Autodesk Fusion 360 part; units mm, degrees
note: some values were not read from the file. Set by a fixed rule: which sketch regions a step uses.
(part 3 of 4)
extrude "Extrude2" add sketch "Sketch2" along normal blind 1.6 contours L4 L5 L6 L7 | L8 L9 L10 L11 | L12 L13 L14 L15 | L16 L17 L18 L19 | L20 L21 L22 L23 | L24 L25 L26 L27 | L28 L29 L30 L31 | L32 L33 L34 L35 | L36 L37 L38 L39 | L40 L41 L42 L43 | L44 L45 L46 L47 | L48 L49 L50 L51 | L52 L53 L54 L55 | L56 L57 L58 L59 | L60 L61 L62 L63 | L64 L65 L66 L67 | L68 L69 L70 L71 | L72 L73 L74 L75 | L76 L77 L78 L79 | L80 L81 L82 L83 | L84 L85 L86 L87 | L88 L89 L90 L91 | L92 L93 L94 L95 | L96 L97 L98 L99 | L100 L101 L102 L103 | L104 L105 L106 L107 | L108 L109 L110 L111 | L112 L113 L114 L115 | L116 L117 L118 L119 | L120 L121 L122 L123 | L124 L125 L126 L127 | L128 L129 L130 L131 | L132 L133 L134 L135 | L136 L137 L138 L139 | L140 L141 L142 L143 | L144 L145 L146 L147 | L148 L149 L150 L151 | L152 L153 L154 L155 | L156 L157 L158 L159 | L160 L161 L162 L163 | L164 L165 L166 L167 | L168 L169 L170 L171 | L172 L173 L174 L175 | L176 L177 L178 L179 | L180 L181 L182 L183 | L184 L185 L186 L187 | L188 L189 L190 L191 | L192 L193 L194 L195 | L196 L197 L198 L199 | L200 L201 L202 L203 | L204 L205 L206 L207 | L208 L209 L210 L211 | L212 L213 L214 L215 | L216 L217 L218 L219 | L220 L221 L222 L223 | L224 L225 L226 L227 | L228 L229 L230 L231 | L232 L233 L234 L235 | L236 L237 L238 L239 | L240 L241 L242 L243 | L244 L245 L246 L247 | L248 L249 L250 L251 | L252 L253 L254 L255 | L256 L257 L258 L259 | L260 L261 L262 L263 | L264 L265 L266 L267 | L268 L269 L270 L271 | L272 L273 L274 L275 | L276 L277 L278 L279 | L280 L281 L282 L283 | L284 L285 L286 L287 | L288 L289 L290 L291 | L292 L293 L294 L295 | L296 L297 L298 L299 | L300 L301 L302 L303 | L304 L305 L306 L307 | L308 L309 L310 L311 | L312 L313 L314 L315 | L316 L317 L318 L319 | L320 L321 L322 L323 | L324 L325 L326 L327 | L328 L329 L330 L331 | L332 L333 L334 L335 | L336 L337 L338 L339 | L340 L341 L342 L343 | L344 L345 L346 L347 | L348 L349 L350 L351 | L352 L353 L354 L355 | L356 L357 L358 L359 | L360 L361 L362 L363 | L364 L365 L366 L367 | L368 L369 L370 L371 | L372 L373 L374 L375 | L376 L377 L378 L379 | L380 L381 L382 L383 | L384 L385 L386 L387 | L388 L389 L390 L391 | L392 L393 L394 L395 | L396 L397 L398 L399 | L400 L401 L402 L403 | L404 L405 L406 L407 | L408 L409 L410 L411 | L412 L413 L414 L415 | L416 L417 L418 L419 | L420 L421 L422 L423 | L424 L425 L426 L427 | L428 L429 L430 L431 | L432 L433 L434 L435 | L436 L437 L438 L439 | L440 L441 L442 L443 | L444 L445 L446 L447 | L448 L449 L450 L451 | L452 L453 L454 L455 | L456 L457 L458 L459 | L460 L461 L462 L463 | L464 L465 L466 L467 | L468 L469 L470 L471 | L472 L473 L474 L475 | L476 L477 L478 L479 | L480 L481 L482 L483 | L484 L485 L486 L487 | L488 L489 L490 L491 | L492 L493 L494 L495 | L496 L497 L498 L499 | L500 L501 L502 L503 | L504 L505 L506 L507 | L508 L509 L510 L511 | L512 L513 L514 L515 | L516 L517 L518 L519 | L520 L521 L522 L523 | L524 L525 L526 L527 | L528 L529 L530 L531 | L532 L533 L534 L535 | L536 L537 L538 L539 | L540 L541 L542 L543 | L544 L545 L546 L547 | L548 L549 L550 L551 | L552 L553 L554 L555 | L556 L557 L558 L559 | L560 L561 L562 L563 | L564 L565 L566 L567 | L568 L569 L570 L571 | L572 L573 L574 L575 | L576 L577 L578 L579 | L580 L581 L582 L583 | L584 L585 L586 L587 | L588 L589 L590 L591 | L592 L593 L594 L595 | L596 L597 L598 L599 | L600 L601 L602 L603 | L604 L605 L606 L607 | L608 L609 L610 L611 | L612 L613 L614 L615 | L616 L617 L618 L619 | L620 L621 L622 L623 | L624 L625 L626 L627 | L628 L629 L630 L631 | L632 L633 L634 L635 | L636 L637 L638 L639 | L640 L641 L642 L643 | L644 L645 L646 L647 | L648 L649 L650 L651 | L652 L653 L654 L655 | L656 L657 L658 L659 | L660 L661 L662 L663 | L664 L665 L666 L667 | L668 L669 L670 L671 | L672 L673 L674 L675 | L676 L677 L678 L679 | L680 L681 L682 L683 | L684 L685 L686 L687 | L688 L689 L690 L691 | L692 L693 L694 L695 | L696 L697 L698 L699 | L700 L701 L702 L703 | L704 L705 L706 L707 | L708 L709 L710 L711 | L712 L713 L714 L715 | L716 L717 L718 L719 | L720 L721 L722 L723 | L724 L725 L726 L727 | L728 L729 L730 L731 | L732 L733 L734 L735 | L736 L737 L738 L739 | L740 L741 L742 L743 | L744 L745 L746 L747 | L748 L749 L750 L751 | L752 L753 L754 L755 | L756 L757 L758 L759 | L760 L761 L762 L763 | L764 L765 L766 L767 | L768 L769 L770 L771 | L772 L773 L774 L775 | L776 L777 L778 L779 | L780 L781 L782 L783 | L784 L785 L786 L787 | L788 L789 L790 L791 | L792 L793 L794 L795 | L796 L797 L798 L799 | L800 L801 L802 L803 | L804 L805 L806 L807 | L808 L809 L810 L811 | L812 L813 L814 L815 | L816 L817 L818 L819 | L820 L821 L822 L823 | L824 L825 L826 L827 | L828 L829 L830 L831 | L832 L833 L834 L835 | L836 L837 L838 L839 | L840 L841 L842 L843 | L844 L845 L846 L847 | L848 L849 L850 L851 | L852 L853 L854 L855 | L856 L857 L858 L859 | L860 L861 L862 L863 | L864 L865 L866 L867 | L868 L869 L870 L871 | L872 L873 L874 L875 | L876 L877 L878 L879 | L880 L881 L882 L883 | L884 L885 L886 L887 | L888 L889 L890 L891 | L892 L893 L894 L895 | L896 L897 L898 L899 | L900 L901 L902 L903 | L904 L905 L906 L907 | L908 L909 L910 L911 | L912 L913 L914 L915 | L916 L917 L918 L919 | L920 L921 L922 L923 | L924 L925 L926 L927 | L928 L929 L930 L931 | L932 L933 L934 L935 | L936 L937 L938 L939 | L940 L941 L942 L943 | L944 L945 L946 L947 | L948 L949 L950 L951 | L952 L953 L954 L955 | L956 L957 L958 L959 | L960 L961 L962 L963 | L964 L965 L966 L967 | L968 L969 L970 L971 | L972 L973 L974 L975 | L976 L977 L978 L979 | L980 L981 L982 L983 | L984 L985 L986 L987 | L988 L989 L990 L991 | L992 L993 L994 L995 | L996 L997 L998 L999 | L1000 L1001 L1002 L1003 | L1004 L1005 L1006 L1007 | L1008 L1009 L1010 L1011 | L1012 L1013 L1014 L1015 | L1016 L1017 L1018 L1019 | L1020 L1021 L1022 L1023 | L1024 L1025 L1026 L1027 bodies 1 in component "LED_Pannel"
extrude "Extrude3" add sketch "Sketch2" along normal blind 1 contours L1028 L1029 L1030 L1031 | L1032 L1033 L1034 L1035 | L1036 L1037 L1038 L1039 | L1040 L1041 L1042 L1043 | L1044 L1045 L1046 L1047 | L1048 L1049 L1050 L1051 | L1052 L1053 L1054 L1055 | L1056 L1057 L1058 L1059 | L1060 L1061 L1062 L1063 | L1064 L1065 L1066 L1067 | L1068 L1069 L1070 L1071 | L1072 L1073 L1074 L1075 | L1076 L1077 L1078 L1079 | L1080 L1081 L1082 L1083 | L1084 L1085 L1086 L1087 | L1088 L1089 L1090 L1091 | L1092 L1093 L1094 L1095 | L1096 L1097 L1098 L1099 | L1100 L1101 L1102 L1103 | L1104 L1105 L1106 L1107 | L1108 L1109 L1110 L1111 | L1112 L1113 L1114 L1115 | L1116 L1117 L1118 L1119 | L1120 L1121 L1122 L1123 | L1124 L1125 L1126 L1127 | L1128 L1129 L1130 L1131 | L1132 L1133 L1134 L1135 | L1136 L1137 L1138 L1139 | L1140 L1141 L1142 L1143 | L1144 L1145 L1146 L1147 | L1148 L1149 L1150 L1151 | L1152 L1153 L1154 L1155 | L1156 L1157 L1158 L1159 | L1160 L1161 L1162 L1163 | L1164 L1165 L1166 L1167 | L1168 L1169 L1170 L1171 | L1172 L1173 L1174 L1175 | L1176 L1177 L1178 L1179 | L1180 L1181 L1182 L1183 | L1184 L1185 L1186 L1187 | L1188 L1189 L1190 L1191 | L1192 L1193 L1194 L1195 | L1196 L1197 L1198 L1199 | L1200 L1201 L1202 L1203 | L1204 L1205 L1206 L1207 | L1208 L1209 L1210 L1211 | L1212 L1213 L1214 L1215 | L1216 L1217 L1218 L1219 | L1220 L1221 L1222 L1223 | L1224 L1225 L1226 L1227 | L1228 L1229 L1230 L1231 | L1232 L1233 L1234 L1235 | L1236 L1237 L1238 L1239 | L1240 L1241 L1242 L1243 | L1244 L1245 L1246 L1247 | L1248 L1249 L1250 L1251 | L1252 L1253 L1254 L1255 | L1256 L1257 L1258 L1259 | L1260 L1261 L1262 L1263 | L1264 L1265 L1266 L1267 | L1268 L1269 L1270 L1271 | L1272 L1273 L1274 L1275 | L1276 L1277 L1278 L1279 | L1280 L1281 L1282 L1283 | L1284 L1285 L1286 L1287 | L1288 L1289 L1290 L1291 | L1292 L1293 L1294 L1295 | L1296 L1297 L1298 L1299 | L1300 L1301 L1302 L1303 | L1304 L1305 L1306 L1307 | L1308 L1309 L1310 L1311 | L1312 L1313 L1314 L1315 | L1316 L1317 L1318 L1319 | L1320 L1321 L1322 L1323 | L1324 L1325 L1326 L1327 | L1328 L1329 L1330 L1331 | L1332 L1333 L1334 L1335 | L1336 L1337 L1338 L1339 | L1340 L1341 L1342 L1343 | L1344 L1345 L1346 L1347 | L1348 L1349 L1350 L1351 | L1352 L1353 L1354 L1355 | L1356 L1357 L1358 L1359 | L1360 L1361 L1362 L1363 | L1364 L1365 L1366 L1367 | L1368 L1369 L1370 L1371 | L1372 L1373 L1374 L1375 | L1376 L1377 L1378 L1379 | L1380 L1381 L1382 L1383 | L1384 L1385 L1386 L1387 | L1388 L1389 L1390 L1391 | L1392 L1393 L1394 L1395 | L1396 L1397 L1398 L1399 | L1400 L1401 L1402 L1403 | L1404 L1405 L1406 L1407 | L1408 L1409 L1410 L1411 | L1412 L1413 L1414 L1415 | L1416 L1417 L1418 L1419 | L1420 L1421 L1422 L1423 | L1424 L1425 L1426 L1427 | L1428 L1429 L1430 L1431 | L1432 L1433 L1434 L1435 | L1436 L1437 L1438 L1439 | L1440 L1441 L1442 L1443 | L1444 L1445 L1446 L1447 | L1448 L1449 L1450 L1451 | L1452 L1453 L1454 L1455 | L1456 L1457 L1458 L1459 | L1460 L1461 L1462 L1463 | L1464 L1465 L1466 L1467 | L1468 L1469 L1470 L1471 | L1472 L1473 L1474 L1475 | L1476 L1477 L1478 L1479 | L1480 L1481 L1482 L1483 | L1484 L1485 L1486 L1487 | L1488 L1489 L1490 L1491 | L1492 L1493 L1494 L1495 | L1496 L1497 L1498 L1499 | L1500 L1501 L1502 L1503 | L1504 L1505 L1506 L1507 | L1508 L1509 L1510 L1511 | L1512 L1513 L1514 L1515 | L1516 L1517 L1518 L1519 | L1520 L1521 L1522 L1523 | L1524 L1525 L1526 L1527 | L1528 L1529 L1530 L1531 | L1532 L1533 L1534 L1535 | L1536 L1537 L1538 L1539 | L1540 L1541 L1542 L1543 | L1544 L1545 L1546 L1547 | L1548 L1549 L1550 L1551 | L1552 L1553 L1554 L1555 | L1556 L1557 L1558 L1559 | L1560 L1561 L1562 L1563 | L1564 L1565 L1566 L1567 | L1568 L1569 L1570 L1571 | L1572 L1573 L1574 L1575 | L1576 L1577 L1578 L1579 | L1580 L1581 L1582 L1583 | L1584 L1585 L1586 L1587 | L1588 L1589 L1590 L1591 | L1592 L1593 L1594 L1595 | L1596 L1597 L1598 L1599 | L1600 L1601 L1602 L1603 | L1604 L1605 L1606 L1607 | L1608 L1609 L1610 L1611 | L1612 L1613 L1614 L1615 | L1616 L1617 L1618 L1619 | L1620 L1621 L1622 L1623 | L1624 L1625 L1626 L1627 | L1628 L1629 L1630 L1631 | L1632 L1633 L1634 L1635 | L1636 L1637 L1638 L1639 | L1640 L1641 L1642 L1643 | L1644 L1645 L1646 L1647 | L1648 L1649 L1650 L1651 | L1652 L1653 L1654 L1655 | L1656 L1657 L1658 L1659 | L1660 L1661 L1662 L1663 | L1664 L1665 L1666 L1667 | L1668 L1669 L1670 L1671 | L1672 L1673 L1674 L1675 | L1676 L1677 L1678 L1679 | L1680 L1681 L1682 L1683 | L1684 L1685 L1686 L1687 | L1688 L1689 L1690 L1691 | L1692 L1693 L1694 L1695 | L1696 L1697 L1698 L1699 | L1700 L1701 L1702 L1703 | L1704 L1705 L1706 L1707 | L1708 L1709 L1710 L1711 | L1712 L1713 L1714 L1715 | L1716 L1717 L1718 L1719 | L1720 L1721 L1722 L1723 | L1724 L1725 L1726 L1727 | L1728 L1729 L1730 L1731 | L1732 L1733 L1734 L1735 | L1736 L1737 L1738 L1739 | L1740 L1741 L1742 L1743 | L1744 L1745 L1746 L1747 | L1748 L1749 L1750 L1751 | L1752 L1753 L1754 L1755 | L1756 L1757 L1758 L1759 | L1760 L1761 L1762 L1763 | L1764 L1765 L1766 L1767 | L1768 L1769 L1770 L1771 | L1772 L1773 L1774 L1775 | L1776 L1777 L1778 L1779 | L1780 L1781 L1782 L1783 | L1784 L1785 L1786 L1787 | L1788 L1789 L1790 L1791 | L1792 L1793 L1794 L1795 | L1796 L1797 L1798 L1799 | L1800 L1801 L1802 L1803 | L1804 L1805 L1806 L1807 | L1808 L1809 L1810 L1811 | L1812 L1813 L1814 L1815 | L1816 L1817 L1818 L1819 | L1820 L1821 L1822 L1823 | L1824 L1825 L1826 L1827 | L1828 L1829 L1830 L1831 | L1832 L1833 L1834 L1835 | L1836 L1837 L1838 L1839 | L1840 L1841 L1842 L1843 | L1844 L1845 L1846 L1847 | L1848 L1849 L1850 L1851 | L1852 L1853 L1854 L1855 | L1856 L1857 L1858 L1859 | L1860 L1861 L1862 L1863 | L1864 L1865 L1866 L1867 | L1868 L1869 L1870 L1871 | L1872 L1873 L1874 L1875 | L1876 L1877 L1878 L1879 | L1880 L1881 L1882 L1883 | L1884 L1885 L1886 L1887 | L1888 L1889 L1890 L1891 | L1892 L1893 L1894 L1895 | L1896 L1897 L1898 L1899 | L1900 L1901 L1902 L1903 | L1904 L1905 L1906 L1907 | L1908 L1909 L1910 L1911 | L1912 L1913 L1914 L1915 | L1916 L1917 L1918 L1919 | L1920 L1921 L1922 L1923 | L1924 L1925 L1926 L1927 | L1928 L1929 L1930 L1931 | L1932 L1933 L1934 L1935 | L1936 L1937 L1938 L1939 | L1940 L1941 L1942 L1943 | L1944 L1945 L1946 L1947 | L1948 L1949 L1950 L1951 | L1952 L1953 L1954 L1955 | L1956 L1957 L1958 L1959 | L1960 L1961 L1962 L1963 | L1964 L1965 L1966 L1967 | L1968 L1969 L1970 L1971 | L1972 L1973 L1974 L1975 | L1976 L1977 L1978 L1979 | L1980 L1981 L1982 L1983 | L1984 L1985 L1986 L1987 bodies 1 in component "LED_Pannel"
sketch "Sketch1 (2)" plane through (0, 0, 0) normal (0, 0, 1) x (1, 0, 0) in component "Diffusion"
  line L0 (0, 0) -> (170, 0)
  line L1 (170, 0) -> (170, 170)
  line L2 (170, 170) -> (0, 170)
  line L3 (0, 170) -> (0, 0)
  dimension "d26" = 170
  constraint horizontal L0
  constraint vertical L1
  constraint horizontal L2
  constraint vertical L3
  constraint coincident L0.start L3.end
  constraint equal L2 L3
  measures "d26" distance of L0.start L2.end
extrude "Extrude1'" add sketch "Sketch1 (2)" along normal blind 3 separate body makes body 2 in component "Diffusion"
sketch "Sketch1 (3)" plane through (0, 0, 0) normal (0, 0, 1) x (1, 0, 0) in component "Backing"
  line L0 (0, 0) -> (170, 0)
  line L1 (170, 0) -> (170, 170)
  line L2 (170, 170) -> (0, 170)
  line L3 (0, 170) -> (0, 0)
  dimension "d26_1" = 170
  constraint horizontal L0
  constraint vertical L1
  constraint horizontal L2
  constraint vertical L3
  constraint coincident L0.start L3.end
  constraint equal L2 L3
  measures "d26_1" distance of L0.start L2.end
extrude "Extrude1''" add sketch "Sketch1 (3)" along normal blind 3 separate body makes body 3 in component "Backing"
sketch "Sketch1 (4)" plane through (0, 0, 0) normal (0, 0, 1) x (1, 0, 0) in component "Side(holes)"
  line L0 (0, 0) -> (180, 0)
  line L1 (180, 0) -> (180, 54)
  line L2 (180, 54) -> (0, 54)
  line L3 (0, 54) -> (0, 0)
  line L4 (175, 54) -> (175, 0) construction
  line L5 (5, 54) -> (5, 0) construction
  line L6 (0, 27) -> (180, 27) construction
  circle A0 centre (5, 43) radius 1.6
  circle A1 centre (5, 11) radius 1.6
  circle A2 centre (175, 43) radius 1.6
  circle A3 centre (175, 11) radius 1.6
  line L7 (5, 48) -> (175, 48) construction
  line L8 (175, 48) -> (175, 51) construction
  line L9 (175, 51) -> (5, 51) construction
  line L10 (5, 51) -> (5, 48) construction
  line L11 (5, 3) -> (175, 3) construction
  line L12 (175, 3) -> (175, 6) construction
  line L13 (175, 6) -> (5, 6) construction
  line L14 (5, 6) -> (5, 3) construction
  line L15 (90, 54) -> (90, 0) construction
  line L16 (10, 36) -> (170, 36) construction
  line L17 (170, 36) -> (170, 48) construction
  line L18 (170, 48) -> (10, 48) construction
  line L19 (10, 48) -> (10, 36) construction
  point P0 (90, 48)
  point P1 (90, 6)
  point P2 (90, 48)
  dimension "d31" = 5
  dimension "d32" = 5
  dimension "d34" = 3.2
  dimension "d36" = 3.2
  dimension "d37" = 3.2
  dimension "d38" = 3.2
  dimension "d68" = 170
  dimension "d69" = 3
  dimension "d70" = 3
  dimension "d71" = 170
  dimension "d72" = 3
  dimension "d73" = 3
  dimension "d74" = 12
  dimension "d75" = 160
  dimension "d76" = 30
  dimension "d77" = 10
  dimension "d78" = 5
  dimension "d79" = 5
  dimension "d80" = 5
  dimension "d81" = 5
  constraint horizontal L0
  constraint vertical L1
  constraint horizontal L2
  constraint vertical L3
  constraint coincident L0.start L3.end
  constraint coincident L2 L4.start
  constraint coincident L0 L4.end
  constraint perpendicular L0 L4
  constraint coincident L2 L5.start
  constraint coincident L0 L5.end
  constraint perpendicular L0 L5
  constraint midpoint L3 L6.start
  constraint midpoint L1 L6.end
  constraint coincident L5 A0.centre
  constraint coincident L5 A1.centre
  constraint coincident L4 A2.centre
  constraint coincident L4 A3.centre
  constraint horizontal L7
  constraint vertical L8
  constraint horizontal L9
  constraint vertical L10
  constraint horizontal L11
  constraint vertical L12
  constraint horizontal L13
  constraint vertical L14
  constraint midpoint L2 L15.start
  constraint midpoint L0 L15.end
  constraint midpoint L7 P2
  constraint midpoint L13 P1
  constraint coincident L15 P1
  constraint coincident L15 P2
  constraint horizontal L16
  constraint vertical L17
  constraint horizontal L18
  constraint vertical L19
  constraint midpoint L18 P2
  constraint coincident P2 P0
  measures "d31" distance of L3 L5
  measures "d32" distance of L1 L4
  measures "d34" diameter of A0
  measures "d36" diameter of A1
  measures "d37" diameter of A2
  measures "d38" diameter of A3
  measures "d68" distance of L7.start L7.end
  measures "d69" distance of L7.start L9.end
  measures "d70" distance of L11.start L13.end
  measures "d71" distance of L12.end L13.end
  measures "d72" distance of L2 L9
  measures "d73" distance of L0 L11
  measures "d74" distance of L16.start L18.end
  measures "d75" distance of L17.end L18.end
  measures "d76" distance of L13 L16
  measures "d77" distance of L3 L19
  measures "d78" distance of A0.centre L7
  measures "d79" distance of A1.centre L13
  measures "d80" distance of A2.centre L7.end
  measures "d81" distance of A3.centre L12.end
extrude "Extrude1'''" add sketch "Sketch1 (4)" along normal blind 10 separate body makes body 4 in component "Side(holes)"
sketch "Sketch2 (2)" plane through (0, 0, 10) normal (0, 0, 1) x (-1, 0, 0) in component "Side(holes)"
  circle A0 centre (-5, -43) radius 1.6 construction
  circle A1 centre (-175, -43) radius 1.6 construction
  circle A2 centre (-5, -11) radius 1.6 construction
  circle A3 centre (-175, -11) radius 1.6 construction
  line L0 (0, -54) -> (0, 0) construction
  line L1 (0, 0) -> (-180, 0) construction
  line L2 (-180, 0) -> (-180, -54) construction
  line L3 (-180, -54) -> (0, -54) construction
  line L4 (-5, -48) -> (-175, -48)
  line L5 (-175, -48) -> (-175, -51)
  line L6 (-175, -51) -> (-5, -51)
  line L7 (-5, -51) -> (-5, -48)
  line L8 (-90, -54) -> (-90, 0) construction
  line L9 (-5, -6) -> (-175, -6)
  line L10 (-175, -6) -> (-175, -3)
  line L11 (-175, -3) -> (-5, -3)
  line L12 (-5, -3) -> (-5, -6)
  line L13 (-89, -48) -> (-91, -48)
  line L14 (-91, -48) -> (-91, -38)
  line L15 (-91, -38) -> (-89, -38)
  line L16 (-89, -38) -> (-89, -48)
  line L17 (-159, -38) -> (-159, -48)
  line L18 (-161, -48) -> (-161, -38)
  line L19 (-161, -38) -> (-159, -38)
  line L20 (-149, -38) -> (-149, -48)
  line L21 (-151, -48) -> (-151, -38)
  line L22 (-151, -38) -> (-149, -38)
  line L23 (-139, -38) -> (-139, -48)
  line L24 (-141, -48) -> (-141, -38)
  line L25 (-141, -38) -> (-139, -38)
  line L26 (-129, -38) -> (-129, -48)
  line L27 (-131, -48) -> (-131, -38)
  line L28 (-131, -38) -> (-129, -38)
  line L29 (-119, -38) -> (-119, -48)
  line L30 (-121, -48) -> (-121, -38)
  line L31 (-121, -38) -> (-119, -38)
  line L32 (-109, -38) -> (-109, -48)
  line L33 (-111, -48) -> (-111, -38)
  line L34 (-111, -38) -> (-109, -38)
  line L35 (-99, -38) -> (-99, -48)
  line L36 (-101, -48) -> (-101, -38)
  line L37 (-101, -38) -> (-99, -38)
  line L38 (-79, -38) -> (-79, -48)
  line L39 (-81, -48) -> (-81, -38)
  line L40 (-81, -38) -> (-79, -38)
  line L41 (-69, -38) -> (-69, -48)
  line L42 (-71, -48) -> (-71, -38)
  line L43 (-71, -38) -> (-69, -38)
  line L44 (-59, -38) -> (-59, -48)
  line L45 (-61, -48) -> (-61, -38)
  line L46 (-61, -38) -> (-59, -38)
  line L47 (-49, -38) -> (-49, -48)
  line L48 (-51, -48) -> (-51, -38)
  line L49 (-51, -38) -> (-49, -38)
  line L50 (-39, -38) -> (-39, -48)
  line L51 (-41, -48) -> (-41, -38)
  line L52 (-41, -38) -> (-39, -38)
  line L53 (-29, -38) -> (-29, -48)
  line L54 (-31, -48) -> (-31, -38)
  line L55 (-31, -38) -> (-29, -38)
  line L56 (-19, -38) -> (-19, -48)
  line L57 (-21, -48) -> (-21, -38)
  line L58 (-21, -38) -> (-19, -38)
  line L59 (-10, -48) -> (-10, -36)
  line L60 (-10, -36) -> (-170, -36)
  line L61 (-170, -36) -> (-170, -48)
  line L62 (-180, -21) -> (0, -21) construction
  line L63 (-10, -36) -> (-10, -6) construction
  line L64 (-170, -36) -> (-170, -6) construction
  circle A4 centre (-25.85, -21) radius 3.85
  circle A5 centre (-44.55, -21) radius 2.85
  circle A6 centre (-65.4, -21) radius 6
  line L65 (-18.35, -28.5) -> (-33.35, -28.5)
  line L66 (-33.35, -28.5) -> (-33.35, -13.5)
  line L67 (-33.35, -13.5) -> (-18.35, -13.5)
  line L68 (-18.35, -13.5) -> (-18.35, -28.5)
  line L69 (-34.55, -31) -> (-54.55, -31)
  line L70 (-54.55, -31) -> (-54.55, -11)
  line L71 (-54.55, -11) -> (-34.55, -11)
  line L72 (-34.55, -11) -> (-34.55, -31)
  line L73 (-57.4, -29) -> (-73.4, -29)
  line L74 (-73.4, -29) -> (-73.4, -13)
  line L75 (-73.4, -13) -> (-57.4, -13)
  line L76 (-57.4, -13) -> (-57.4, -29)
  line L77 (-73.4, -29) -> (-57.4, -13) construction
  line L78 (-54.55, -31) -> (-34.55, -11) construction
  line L79 (-33.35, -28.5) -> (-18.35, -13.5) construction
  point P0 (-90, -51)
  point P1 (-90, -6)
  point P2 (-90, -38)
  point P3 (-90, -48)
  point P4 (-90, -38)
  point P5 (-10, -21)
  point P6 (-10, -21)
  point P7 (-170, -21)
  point P8 (-29.7, -21)
  point P9 (-41.7, -21)
  point P10 (-47.4, -21)
  point P11 (-59.4, -21)
  point P12 (-71.4, -21)
  point P13 (-22, -21)
  point P14 (-25.85, -21)
  point P15 (-44.55, -21)
  point P16 (-65.4, -21)
  dimension "d44" = 170
  dimension "d45" = 3
  dimension "d46" = 3
  dimension "d47" = 170
  dimension "d48" = 3
  dimension "d49" = 3
  dimension "d50" = 2
  dimension "d51" = 10
  dimension "d54" = 10
  dimension "d55" = 0
  dimension "d83" = 7.7
  dimension "d84" = 5.7
  dimension "d85" = 12
  dimension "d87" = 12
  dimension "d88" = 12
  dimension "d89" = 12
  dimension "d93" = 16
  dimension "d94" = 20
  dimension "d95" = 15
  constraint horizontal L4
  constraint vertical L5
  constraint horizontal L6
  constraint vertical L7
  constraint midpoint L3 L8.start
  constraint midpoint L1 L8.end
  constraint midpoint L6 P0
  constraint coincident L8 P0
  constraint horizontal L9
  constraint vertical L10
  constraint horizontal L11
  constraint vertical L12
  constraint midpoint L9 P1
  constraint coincident L8 P1
  constraint horizontal L13
  constraint vertical L14
  constraint horizontal L15
  constraint vertical L16
  constraint midpoint L15 P4
  constraint coincident L8 P4
  constraint midpoint L13 P3
  constraint coincident L4 P3
  constraint coincident P4 P2
  constraint coincident L2 L62.start
  constraint coincident L0 L62.end
  constraint perpendicular L0 L62
  constraint coincident L59.end L60.start
  constraint coincident L9 L63.end
  constraint perpendicular L9 L63
  constraint midpoint L63 P6
  constraint coincident L62 P6
  constraint coincident P6 P5
  constraint coincident L60.end L61.start
  constraint coincident L9 L64.end
  constraint perpendicular L9 L64
  constraint midpoint L64 P7
  constraint coincident L62 P14
  constraint coincident L62 P15
  constraint coincident L62 P16
  constraint coincident A4 P8
  constraint coincident L62 P8
  constraint coincident A5 P9
  constraint coincident L62 P9
  constraint coincident A5 P10
  constraint coincident L62 P10
  constraint coincident A6 P11
  constraint coincident L62 P11
  constraint coincident A6 P12
  constraint coincident L62 P12
  constraint coincident A4 P13
  constraint coincident L62 P13
  constraint horizontal L65
  constraint vertical L66
  constraint horizontal L67
  constraint vertical L68
  constraint horizontal L69
  constraint vertical L70
  constraint horizontal L71
  constraint vertical L72
  constraint horizontal L73
  constraint vertical L74
  constraint horizontal L75
  constraint vertical L76
  constraint midpoint L79 P14
  constraint midpoint L78 P15
  constraint midpoint L77 P16
  constraint coincident P14 A4.centre
  constraint coincident P15 A5.centre
  constraint coincident P16 A6.centre
  constraint equal L65 L68
  constraint equal L69 L72
  constraint equal L73 L76
  measures "d44" distance of L4.start L4.end
  measures "d45" distance of L4.start L6.end
  measures "d46" distance of L3 L6
  measures "d47" distance of L9.start L9.end
  measures "d48" distance of L9.start L11.end
  measures "d49" distance of L1 L11
  measures "d50" distance of L13.start L13.end
  measures "d51" distance of L13.start L15.end
  measures "d83" diameter of A4
  measures "d84" diameter of A5
  measures "d85" diameter of A6
  measures "d87" distance of P6 P13
  measures "d88" distance of P8 P9
  measures "d89" distance of P10 P11
  measures "d93" distance of L74.end L75.end
  measures "d94" distance of L70.end L71.end
  measures "d95" distance of L66.end L67.end
extrude "Extrude2'" cut sketch "Sketch2 (2)" against normal blind 5 contours L4 L5 L6 L7 L13 | L4 L56 L57 L58 | L4 L53 L54 L55 | L4 L17 L18 L19 | L4 L50 L51 L52 | L4 L20 L21 L22 | L4 L47 L48 L49 | L4 L23 L24 L25 | L4 L44 L45 L46 | L4 L26 L27 L28 | L4 L41 L42 L43 | L4 L29 L30 L31 | L4 L38 L39 L40 | L4 L32 L33 L34 | L4 L13 L14 L15 L16 | L4 L35 L36 L37 | L9 L10 L11 L12 bodies 4 in component "Side(holes)"
chamfer "Chamfer2" distance 1 angle 45 66 edges at (5, 49.5, 10) (12, 48, 10) (19, 43, 10) (21, 43, 10) (20, 38, 10) (25, 48, 10) (29, 43, 10) (31, 43, 10) (30, 38, 10) (35, 48, 10) (41, 43, 10) (39, 43, 10) (40, 38, 10) (51, 43, 10) (49, 43, 10) (45, 48, 10) (50, 38, 10) (61, 43, 10) (59, 43, 10) (55, 48, 10) (60, 38, 10) (65, 48, 10) (69, 43, 10) (71, 43, 10) (70, 38, 10) (79, 43, 10) (81, 43, 10) (75, 48, 10) (80, 38, 10) (85, 48, 10) (89, 43, 10) (91, 43, 10) (90, 38, 10) (95, 48, 10) (99, 43, 10) (101, 43, 10) (100, 38, 10) (105, 48, 10) (109, 43, 10) (111, 43, 10) (110, 38, 10) (115, 48, 10) (119, 43, 10) (121, 43, 10) (120, 38, 10) (125, 48, 10) (129, 43, 10) (131, 43, 10) (130, 38, 10) (135, 48, 10) (139, 43, 10) (141, 43, 10) (140, 38, 10) (145, 48, 10) (149, 43, 10) (150, 38, 10) (151, 43, 10) (155, 48, 10) (159, 43, 10) (161, 43, 10) (160, 38, 10) (168, 48, 10) (175, 49.5, 10) (5, 4.5, 10) (90, 6, 10) (175, 4.5, 10) on bodies 4 in component "Side(holes)"
extrude "Extrude3'" cut sketch "Sketch2 (2)" against normal blind 10 contours A4 | A5 | A6 bodies 4 in component "Side(holes)"
extrude "Extrude4" cut sketch "Sketch2 (2)" against normal blind 8 contours L65 L66 L67 L68 | L69 L70 L71 L72 | L73 L74 L75 L76 bodies 4 in component "Side(holes)"
sketch "Sketch1 (5)" plane through (0, 0, 0) normal (0, 0, 1) x (1, 0, 0) in component "Side(no holes)"
  line L0 (0, 0) -> (180, 0)
  line L1 (180, 0) -> (180, 54)
  line L2 (180, 54) -> (0, 54)
  line L3 (0, 54) -> (0, 0)
  line L4 (175, 54) -> (175, 0) construction
  line L5 (5, 54) -> (5, 0) construction
  line L6 (0, 27) -> (180, 27) construction
  circle A0 centre (5, 43) radius 1.6
  circle A1 centre (5, 11) radius 1.6
  circle A2 centre (175, 43) radius 1.6
  circle A3 centre (175, 11) radius 1.6
  line L7 (5, 48) -> (175, 48) construction
  line L8 (175, 48) -> (175, 51) construction
  line L9 (175, 51) -> (5, 51) construction
  line L10 (5, 51) -> (5, 48) construction
  line L11 (5, 3) -> (175, 3) construction
  line L12 (175, 3) -> (175, 6) construction
  line L13 (175, 6) -> (5, 6) construction
  line L14 (5, 6) -> (5, 3) construction
  line L15 (90, 54) -> (90, 0) construction
  line L16 (10, 36) -> (170, 36) construction
  line L17 (170, 36) -> (170, 48) construction
  line L18 (170, 48) -> (10, 48) construction
  line L19 (10, 48) -> (10, 36) construction
  point P0 (90, 48)
  point P1 (90, 6)
  point P2 (90, 48)
  dimension "d31_1" = 5
  dimension "d32_1" = 5
  dimension "d34_1" = 3.2
  dimension "d36_1" = 3.2
  dimension "d37_1" = 3.2
  dimension "d38_1" = 3.2
  dimension "d68_1" = 170
  dimension "d69_1" = 3
  dimension "d70_1" = 3
  dimension "d71_1" = 170
  dimension "d72_1" = 3
  dimension "d73_1" = 3
  dimension "d74_1" = 12
  dimension "d75_1" = 160
  dimension "d76_1" = 30
  dimension "d77_1" = 10
  dimension "d78_1" = 5
  dimension "d79_1" = 5
  dimension "d80_1" = 5
  dimension "d81_1" = 5
  constraint horizontal L0
  constraint vertical L1
  constraint horizontal L2
  constraint vertical L3
  constraint coincident L0.start L3.end
  constraint coincident L2 L4.start
  constraint coincident L0 L4.end
  constraint perpendicular L0 L4
  constraint coincident L2 L5.start
  constraint coincident L0 L5.end
  constraint perpendicular L0 L5
  constraint midpoint L3 L6.start
  constraint midpoint L1 L6.end
  constraint coincident L5 A0.centre
  constraint coincident L5 A1.centre
  constraint coincident L4 A2.centre
  constraint coincident L4 A3.centre
  constraint horizontal L7
  constraint vertical L8
  constraint horizontal L9
  constraint vertical L10
  constraint horizontal L11
  constraint vertical L12
  constraint horizontal L13
  constraint vertical L14
  constraint midpoint L2 L15.start
  constraint midpoint L0 L15.end
  constraint midpoint L7 P2
  constraint midpoint L13 P1
  constraint coincident L15 P1
  constraint coincident L15 P2
  constraint horizontal L16
  constraint vertical L17
  constraint horizontal L18
  constraint vertical L19
  constraint midpoint L18 P2
  constraint coincident P2 P0
  measures "d31_1" distance of L3 L5
  measures "d32_1" distance of L1 L4
  measures "d34_1" diameter of A0
  measures "d36_1" diameter of A1
  measures "d37_1" diameter of A2
  measures "d38_1" diameter of A3
  measures "d68_1" distance of L7.start L7.end
  measures "d69_1" distance of L7.start L9.end
  measures "d70_1" distance of L11.start L13.end
  measures "d71_1" distance of L12.end L13.end
  measures "d72_1" distance of L2 L9
  measures "d73_1" distance of L0 L11
  measures "d74_1" distance of L16.start L18.end
  measures "d75_1" distance of L17.end L18.end
  measures "d76_1" distance of L13 L16
  measures "d77_1" distance of L3 L19
  measures "d78_1" distance of A0.centre L7
  measures "d79_1" distance of A1.centre L13
  measures "d80_1" distance of A2.centre L7.end
  measures "d81_1" distance of A3.centre L12.end
extrude "Extrude1''''" add sketch "Sketch1 (5)" along normal blind 10 separate body makes body 5 in component "Side(no holes)"
sketch "Sketch2 (3)" plane through (0, 0, 10) normal (0, 0, 1) x (-1, 0, 0) in component "Side(no holes)"
  circle A0 centre (-5, -43) radius 1.6 construction
  circle A1 centre (-175, -43) radius 1.6 construction
  circle A2 centre (-5, -11) radius 1.6 construction
  circle A3 centre (-175, -11) radius 1.6 construction
  line L0 (0, -54) -> (0, 0) construction
  line L1 (0, 0) -> (-180, 0) construction
  line L2 (-180, 0) -> (-180, -54) construction
  line L3 (-180, -54) -> (0, -54) construction
  line L4 (-5, -48) -> (-175, -48)
  line L5 (-175, -48) -> (-175, -51)
  line L6 (-175, -51) -> (-5, -51)
  line L7 (-5, -51) -> (-5, -48)
  line L8 (-90, -54) -> (-90, 0) construction
  line L9 (-5, -6) -> (-175, -6)
  line L10 (-175, -6) -> (-175, -3)
  line L11 (-175, -3) -> (-5, -3)
  line L12 (-5, -3) -> (-5, -6)
  line L13 (-89, -48) -> (-91, -48)
  line L14 (-91, -48) -> (-91, -38)
  line L15 (-91, -38) -> (-89, -38)
  line L16 (-89, -38) -> (-89, -48)
  line L17 (-159, -38) -> (-159, -48)
  line L18 (-161, -48) -> (-161, -38)
  line L19 (-161, -38) -> (-159, -38)
  line L20 (-149, -38) -> (-149, -48)
  line L21 (-151, -48) -> (-151, -38)
  line L22 (-151, -38) -> (-149, -38)
  line L23 (-139, -38) -> (-139, -48)
  line L24 (-141, -48) -> (-141, -38)
  line L25 (-141, -38) -> (-139, -38)
  line L26 (-129, -38) -> (-129, -48)
  line L27 (-131, -48) -> (-131, -38)
  line L28 (-131, -38) -> (-129, -38)
  line L29 (-119, -38) -> (-119, -48)
  line L30 (-121, -48) -> (-121, -38)
  line L31 (-121, -38) -> (-119, -38)
  line L32 (-109, -38) -> (-109, -48)
  line L33 (-111, -48) -> (-111, -38)
  line L34 (-111, -38) -> (-109, -38)
  line L35 (-99, -38) -> (-99, -48)
  line L36 (-101, -48) -> (-101, -38)
  line L37 (-101, -38) -> (-99, -38)
  line L38 (-79, -38) -> (-79, -48)
  line L39 (-81, -48) -> (-81, -38)
  line L40 (-81, -38) -> (-79, -38)
  line L41 (-69, -38) -> (-69, -48)
  line L42 (-71, -48) -> (-71, -38)
  line L43 (-71, -38) -> (-69, -38)
  line L44 (-59, -38) -> (-59, -48)
  line L45 (-61, -48) -> (-61, -38)
  line L46 (-61, -38) -> (-59, -38)
  line L47 (-49, -38) -> (-49, -48)
  line L48 (-51, -48) -> (-51, -38)
  line L49 (-51, -38) -> (-49, -38)
  line L50 (-39, -38) -> (-39, -48)
  line L51 (-41, -48) -> (-41, -38)
  line L52 (-41, -38) -> (-39, -38)
  line L53 (-29, -38) -> (-29, -48)
  line L54 (-31, -48) -> (-31, -38)
  line L55 (-31, -38) -> (-29, -38)
  line L56 (-19, -38) -> (-19, -48)
  line L57 (-21, -48) -> (-21, -38)
  line L58 (-21, -38) -> (-19, -38)
  line L59 (-10, -48) -> (-10, -36)
  line L60 (-10, -36) -> (-170, -36)
  line L61 (-170, -36) -> (-170, -48)
  line L62 (-180, -21) -> (0, -21) construction
  line L63 (-10, -36) -> (-10, -6) construction
  line L64 (-170, -36) -> (-170, -6) construction
  circle A4 centre (-25.85, -21) radius 3.85
  circle A5 centre (-44.55, -21) radius 2.85
  circle A6 centre (-70.4, -21) radius 11
  circle A7 centre (-99.4, -21) radius 6
  line L65 (-18.35, -28.5) -> (-33.35, -28.5)
  line L66 (-33.35, -28.5) -> (-33.35, -13.5)
  line L67 (-33.35, -13.5) -> (-18.35, -13.5)
  line L68 (-18.35, -13.5) -> (-18.35, -28.5)
  line L69 (-34.55, -31) -> (-54.55, -31)
  line L70 (-54.55, -31) -> (-54.55, -11) construction
  line L71 (-54.55, -11) -> (-34.55, -11)
  line L72 (-34.55, -11) -> (-34.55, -31)
  line L73 (-55.4, -36) -> (-85.4, -36)
  line L74 (-85.4, -36) -> (-85.4, -6)
  line L75 (-85.4, -6) -> (-55.4, -6)
  line L76 (-55.4, -6) -> (-55.4, -36)
  line L77 (-91.4, -29) -> (-107.4, -29)
  line L78 (-107.4, -29) -> (-107.4, -13)
  line L79 (-107.4, -13) -> (-91.4, -13)
  line L80 (-91.4, -13) -> (-91.4, -29)
  line L81 (-107.4, -29) -> (-91.4, -13) construction
  line L82 (-85.4, -36) -> (-55.4, -6) construction
  line L83 (-54.55, -31) -> (-34.55, -11) construction
  line L84 (-33.35, -28.5) -> (-18.35, -13.5) construction
  line L85 (-54.55, -31) -> (-55.4, -31)
  line L86 (-54.55, -11) -> (-55.4, -11)
  point P0 (-90, -51)
  point P1 (-90, -6)
  point P2 (-90, -38)
  point P3 (-90, -48)
  point P4 (-90, -38)
  point P5 (-10, -21)
  point P6 (-10, -21)
  point P7 (-170, -21)
  point P8 (-29.7, -21)
  point P9 (-41.7, -21)
  point P10 (-47.4, -21)
  point P11 (-59.4, -21)
  point P12 (-81.4, -21)
  point P13 (-93.4, -21)
  point P14 (-22, -21)
  point P15 (-25.85, -21)
  point P16 (-44.55, -21)
  point P17 (-70.4, -21)
  point P18 (-99.4, -21)
  dimension "d44_1" = 170
  dimension "d45_1" = 3
  dimension "d46_1" = 3
  dimension "d47_1" = 170
  dimension "d48_1" = 3
  dimension "d49_1" = 3
  dimension "d50_1" = 2
  dimension "d51_1" = 10
  dimension "d54_1" = 10
  dimension "d55_1" = 0
  dimension "d83_1" = 7.7
  dimension "d84_1" = 5.7
  dimension "d85_1" = 22
  dimension "d86_1" = 12
  dimension "d87_1" = 12
  dimension "d88_1" = 12
  dimension "d89_1" = 12
  dimension "d90_1" = 12
  dimension "d92_1" = 16
  dimension "d93_1" = 30
  dimension "d94_1" = 20
  dimension "d95_1" = 15
  constraint horizontal L4
  constraint vertical L5
  constraint horizontal L6
  constraint vertical L7
  constraint midpoint L3 L8.start
  constraint midpoint L1 L8.end
  constraint midpoint L6 P0
  constraint coincident L8 P0
  constraint horizontal L9
  constraint vertical L10
  constraint horizontal L11
  constraint vertical L12
  constraint midpoint L9 P1
  constraint coincident L8 P1
  constraint horizontal L13
  constraint vertical L14
  constraint horizontal L15
  constraint vertical L16
  constraint midpoint L15 P4
  constraint coincident L8 P4
  constraint midpoint L13 P3
  constraint coincident L4 P3
  constraint coincident P4 P2
  constraint coincident L2 L62.start
  constraint coincident L0 L62.end
  constraint perpendicular L0 L62
  constraint coincident L59.end L60.start
  constraint coincident L9 L63.end
  constraint perpendicular L9 L63
  constraint midpoint L63 P6
  constraint coincident L62 P6
  constraint coincident P6 P5
  constraint coincident L60.end L61.start
  constraint coincident L9 L64.end
  constraint perpendicular L9 L64
  constraint midpoint L64 P7
  constraint coincident L62 P15
  constraint coincident L62 P16
  constraint coincident L62 P17
  constraint coincident L62 P18
  constraint coincident A4 P8
  constraint coincident L62 P8
  constraint coincident A5 P9
  constraint coincident L62 P9
  constraint coincident A5 P10
  constraint coincident L62 P10
  constraint coincident A6 P11
  constraint coincident L62 P11
  constraint coincident A6 P12
  constraint coincident L62 P12
  constraint coincident A7 P13
  constraint coincident L62 P13
  constraint coincident A4 P14
  constraint coincident L62 P14
  constraint horizontal L65
  constraint vertical L66
  constraint horizontal L67
  constraint vertical L68
  constraint horizontal L69
  constraint vertical L70
  constraint horizontal L71
  constraint vertical L72
  constraint horizontal L73
  constraint vertical L74
  constraint horizontal L75
  constraint vertical L76
  constraint horizontal L77
  constraint vertical L78
  constraint horizontal L79
  constraint vertical L80
  constraint midpoint L84 P15
  constraint midpoint L83 P16
  constraint midpoint L82 P17
  constraint midpoint L81 P18
  constraint coincident P15 A4.centre
  constraint coincident P16 A5.centre
  constraint coincident P17 A6.centre
  constraint coincident P18 A7.centre
  constraint equal L65 L68
  constraint equal L69 L72
  constraint equal L73 L76
  constraint equal L77 L80
  constraint coincident L76 L85.end
  constraint perpendicular L76 L85
  constraint coincident L76 L86.end
  constraint perpendicular L76 L86
  measures "d44_1" distance of L4.start L4.end
  measures "d45_1" distance of L4.start L6.end
  measures "d46_1" distance of L3 L6
  measures "d47_1" distance of L9.start L9.end
  measures "d48_1" distance of L9.start L11.end
  measures "d49_1" distance of L1 L11
  measures "d50_1" distance of L13.start L13.end
  measures "d51_1" distance of L13.start L15.end
  measures "d83_1" diameter of A4
  measures "d84_1" diameter of A5
  measures "d85_1" diameter of A6
  measures "d86_1" diameter of A7
  measures "d87_1" distance of P6 P14
  measures "d88_1" distance of P8 P9
  measures "d89_1" distance of P10 P11
  measures "d90_1" distance of P12 P13
  measures "d92_1" distance of L78.end L79.end
  measures "d93_1" distance of L74.end L75.end
  measures "d94_1" distance of L70.end L71.end
  measures "d95_1" distance of L66.end L67.end
extrude "Extrude2''" cut sketch "Sketch2 (3)" against normal blind 5 contours L4 L5 L6 L7 L13 | L4 L56 L57 L58 | L4 L53 L54 L55 | L9 L10 L11 L12 L75 | L4 L17 L18 L19 | L4 L50 L51 L52 | L4 L20 L21 L22 | L4 L47 L48 L49 | L4 L23 L24 L25 | L4 L44 L45 L46 | L4 L26 L27 L28 | L4 L41 L42 L43 | L4 L29 L30 L31 | L4 L38 L39 L40 | L4 L32 L33 L34 | L4 L13 L14 L15 L16 | L4 L35 L36 L37 bodies 5 in component "Side(no holes)"
chamfer "Chamfer2'" distance 1 angle 45 66 edges at (5, 49.5, 10) (12, 48, 10) (19, 43, 10) (21, 43, 10) (20, 38, 10) (25, 48, 10) (29, 43, 10) (31, 43, 10) (30, 38, 10) (35, 48, 10) (41, 43, 10) (39, 43, 10) (40, 38, 10) (51, 43, 10) (49, 43, 10) (45, 48, 10) (50, 38, 10) (61, 43, 10) (59, 43, 10) (55, 48, 10) (60, 38, 10) (65, 48, 10) (69, 43, 10) (71, 43, 10) (70, 38, 10) (79, 43, 10) (81, 43, 10) (75, 48, 10) (80, 38, 10) (85, 48, 10) (89, 43, 10) (91, 43, 10) (90, 38, 10) (95, 48, 10) (99, 43, 10) (101, 43, 10) (100, 38, 10) (105, 48, 10) (109, 43, 10) (111, 43, 10) (110, 38, 10) (115, 48, 10) (119, 43, 10) (121, 43, 10) (120, 38, 10) (125, 48, 10) (129, 43, 10) (131, 43, 10) (130, 38, 10) (135, 48, 10) (139, 43, 10) (141, 43, 10) (140, 38, 10) (145, 48, 10) (149, 43, 10) (150, 38, 10) (151, 43, 10) (155, 48, 10) (159, 43, 10) (161, 43, 10) (160, 38, 10) (168, 48, 10) (175, 49.5, 10) (5, 4.5, 10) (90, 6, 10) (175, 4.5, 10) on bodies 5 in component "Side(no holes)"
sketch "Sketch1 (6)" plane through (0, 0, 0) normal (0, 0, 1) x (1, 0, 0) in component "Top/Bottom"
  line L0 (0, 0) -> (160, 0)
  line L1 (160, 0) -> (160, 54)
  line L2 (160, 54) -> (0, 54)
  line L3 (0, 54) -> (0, 0)
  line L4 (0, 51) -> (160, 51) construction
  line L5 (160, 51) -> (160, 48) construction
  line L6 (160, 48) -> (0, 48) construction
  line L7 (0, 48) -> (0, 51) construction
  line L8 (0, 3) -> (160, 3) construction
  line L9 (160, 3) -> (160, 6) construction
  line L10 (160, 6) -> (0, 6) construction
  line L11 (0, 6) -> (0, 3) construction
  line L12 (10, 48) -> (150, 48) construction
  line L13 (150, 48) -> (150, 38) construction
  line L14 (150, 38) -> (10, 38) construction
  line L15 (10, 38) -> (10, 48) construction
  line L16 (0, 38) -> (160, 38) construction
  line L17 (160, 38) -> (160, 36) construction
  line L18 (160, 36) -> (0, 36) construction
  line L19 (0, 36) -> (0, 38) construction
  line L20 (80, 54) -> (80, 0) construction
  point P0 (80, 51)
  point P1 (80, 48)
  point P2 (80, 38)
  point P3 (80, 38)
  point P4 (80, 6)
  dimension "d101" = 160
  dimension "d102" = 3
  dimension "d103" = 3
  dimension "d104" = 10
  dimension "d105" = 2
  dimension "d106" = 140
  dimension "d107" = 30
  dimension "d108" = 3
  dimension "d109" = 3
  constraint horizontal L0
  constraint vertical L1
  constraint horizontal L2
  constraint vertical L3
  constraint coincident L0.start L3.end
  constraint horizontal L4
  constraint vertical L5
  constraint horizontal L6
  constraint vertical L7
  constraint horizontal L8
  constraint vertical L9
  constraint horizontal L10
  constraint vertical L11
  constraint horizontal L12
  constraint vertical L13
  constraint horizontal L14
  constraint vertical L15
  constraint horizontal L16
  constraint vertical L17
  constraint horizontal L18
  constraint vertical L19
  constraint midpoint L2 L20.start
  constraint midpoint L0 L20.end
  constraint midpoint L4 P0
  constraint midpoint L12 P1
  constraint midpoint L16 P3
  constraint midpoint L14 P3
  constraint coincident L20 P0
  constraint coincident P3 P2
  constraint midpoint L10 P4
  constraint coincident L20 P4
  constraint coincident L3 L4.start
  constraint coincident L20 P3
  constraint coincident L6 P1
  constraint coincident L3 L18.end
  constraint coincident L3 L8.start
  measures "d101" distance of L17 L19
  measures "d102" distance of L2 L4
  measures "d103" distance of L4 L6
  measures "d104" distance of L12.start L14.end
  measures "d105" distance of L16.start L18.end
  measures "d106" distance of L13 L15
  measures "d107" distance of L10 L18
  measures "d108" distance of L8 L10
  measures "d109" distance of L0 L8
extrude "Extrude1'''''" add sketch "Sketch1 (6)" along normal blind 10 separate body makes body 6 in component "Top/Bottom"
sketch "Sketch2 (4)" plane through (0, 0, 10) normal (0, 0, 1) x (-1, 0, 0) in component "Top/Bottom"
  line L0 (0, -54) -> (0, 0)
  line L1 (0, 0) -> (-160, 0)
  line L2 (-160, 0) -> (-160, -54)
  line L3 (-160, -54) -> (0, -54)
  line L4 (0, -3) -> (-160, -3)
  line L5 (-160, -6) -> (0, -6)
  line L6 (-160, -48) -> (0, -48)
  line L7 (0, -51) -> (-160, -51)
  line L8 (-79, -48) -> (-81, -48)
  line L9 (-81, -48) -> (-81, -38)
  line L10 (-81, -38) -> (-79, -38)
  line L11 (-79, -38) -> (-79, -48)
  line L12 (-80, -54) -> (-80, 0)
  line L13 (-149, -38) -> (-149, -48)
  line L14 (-151, -48) -> (-151, -38)
  line L15 (-151, -38) -> (-149, -38)
  line L16 (-139, -38) -> (-139, -48)
  line L17 (-141, -48) -> (-141, -38)
  line L18 (-141, -38) -> (-139, -38)
  line L19 (-129, -38) -> (-129, -48)
  line L20 (-131, -48) -> (-131, -38)
  line L21 (-131, -38) -> (-129, -38)
  line L22 (-119, -38) -> (-119, -48)
  line L23 (-121, -48) -> (-121, -38)
  line L24 (-121, -38) -> (-119, -38)
  line L25 (-109, -38) -> (-109, -48)
  line L26 (-111, -48) -> (-111, -38)
  line L27 (-111, -38) -> (-109, -38)
  line L28 (-99, -38) -> (-99, -48)
  line L29 (-101, -48) -> (-101, -38)
  line L30 (-101, -38) -> (-99, -38)
  line L31 (-89, -38) -> (-89, -48)
  line L32 (-91, -48) -> (-91, -38)
  line L33 (-91, -38) -> (-89, -38)
  line L34 (-69, -38) -> (-69, -48)
  line L35 (-71, -48) -> (-71, -38)
  line L36 (-71, -38) -> (-69, -38)
  line L37 (-59, -38) -> (-59, -48)
  line L38 (-61, -48) -> (-61, -38)
  line L39 (-61, -38) -> (-59, -38)
  line L40 (-49, -38) -> (-49, -48)
  line L41 (-51, -48) -> (-51, -38)
  line L42 (-51, -38) -> (-49, -38)
  line L43 (-39, -38) -> (-39, -48)
  line L44 (-41, -48) -> (-41, -38)
  line L45 (-41, -38) -> (-39, -38)
  line L46 (-29, -38) -> (-29, -48)
  line L47 (-31, -48) -> (-31, -38)
  line L48 (-31, -38) -> (-29, -38)
  line L49 (-19, -38) -> (-19, -48)
  line L50 (-21, -48) -> (-21, -38)
  line L51 (-21, -38) -> (-19, -38)
  line L52 (-9, -38) -> (-9, -48)
  line L53 (-11, -48) -> (-11, -38)
  line L54 (-11, -38) -> (-9, -38)
  point P0 (-80, -48)
  dimension "d112" = 2
  dimension "d113" = 10
  dimension "d116" = 10
  dimension "d117" = 0
  constraint horizontal L8
  constraint vertical L9
  constraint horizontal L10
  constraint vertical L11
  constraint midpoint L8 P0
  constraint coincident P0 L12
  constraint coincident L6 P0
  measures "d112" distance of L8.start L8.end
  measures "d113" distance of L8.start L10.end
extrude "Extrude2'''" cut sketch "Sketch2 (4)" against normal blind 5 contours L0 L6 L7 L8 L12 | L2 L6 L7 L8 L12 | L0 L4 L5 L12 | L6 L52 L53 L54 | L6 L8 L10 L11 L12 | L6 L8 L9 L10 L12 | L2 L4 L5 L12 | L6 L49 L50 L51 | L6 L13 L14 L15 | L6 L31 L32 L33 | L6 L34 L35 L36 | L6 L46 L47 L48 | L6 L16 L17 L18 | L6 L28 L29 L30 | L6 L37 L38 L39 | L6 L43 L44 L45 | L6 L19 L20 L21 | L6 L25 L26 L27 | L6 L40 L41 L42 | L6 L22 L23 L24 bodies 6 in component "Top/Bottom"
chamfer "Chamfer1" distance 1 angle 45 62 edges at (155.5, 48, 10) (151, 43, 10) (150, 38, 10) (145, 48, 10) (141, 43, 10) (140, 38, 10) (139, 43, 10) (131, 43, 10) (130, 38, 10) (129, 43, 10) (135, 48, 10) (125, 48, 10) (121, 43, 10) (120, 38, 10) (119, 43, 10) (115, 48, 10) (111, 43, 10) (110, 38, 10) (109, 43, 10) (105, 48, 10) (101, 43, 10) (99, 43, 10) (100, 38, 10) (91, 43, 10) (95, 48, 10) (89, 43, 10) (90, 38, 10) (81, 43, 10) (79, 43, 10) (80, 38, 10) (75, 48, 10) (85, 48, 10) (69, 43, 10) (71, 43, 10) (70, 38, 10) (61, 43, 10) (59, 43, 10) (60, 38, 10) (51, 43, 10) (49, 43, 10) (50, 38, 10) (55, 48, 10) (65, 48, 10) (45, 48, 10) (41, 43, 10) (40, 38, 10) (39, 43, 10) (35, 48, 10) (29, 43, 10) (31, 43, 10) (30, 38, 10) (21, 43, 10) (20, 38, 10) (19, 43, 10) (11, 43, 10) (10, 38, 10) (9, 43, 10) (15, 48, 10) (4.5, 48, 10) (25, 48, 10) (80, 6, 10) (149, 43, 10) on bodies 6 in component "Top/Bottom"
sketch "Sketch3" plane through (0, 0, 0) normal (-1, 0, 0) x (0, -1, 0) in component "Top/Bottom"
  line L0 (-6, 9) -> (-7, 10)
  line L1 (-7, 10) -> (-47, 10)
  line L2 (-47, 10) -> (-48, 9)
  line L3 (-48, 9) -> (-48, 5)
  line L4 (-48, 5) -> (-51, 5)
  line L5 (-51, 5) -> (-51, 10)
  line L6 (-51, 10) -> (-54, 10)
  line L7 (-54, 10) -> (-54, 0)
  line L8 (-54, 0) -> (0, 0)
  line L9 (0, 0) -> (0, 10)
  line L10 (0, 10) -> (-3, 10)
  line L11 (-3, 10) -> (-3, 5)
  line L12 (-3, 5) -> (-6, 5)
  line L13 (-6, 5) -> (-6, 9)
  line L14 (-48, 5) -> (-6, 5) construction
  circle A0 centre (-43, 5) radius 1.85
  circle A1 centre (-11, 5) radius 1.85
  circle A2 centre (-43, 5) radius 1.6
  circle A3 centre (-11, 5) radius 1.6
  dimension "d121" = 3.7
  dimension "d122" = 3.7
  dimension "d123" = 5
  dimension "d124" = 5
  dimension "d127" = 3.2
  dimension "d128" = 3.2
  constraint coincident L3.end L4.start
  constraint coincident L12.end L13.start
  constraint coincident L14 A0.centre
  constraint coincident L14 A1.centre
  constraint concentric A0 A2
  constraint concentric A1 A3
  measures "d121" diameter of A0
  measures "d122" diameter of A1
  measures "d123" distance of L3.end A0.centre
  measures "d124" distance of L12.end A1.centre
  measures "d127" diameter of A2
  measures "d128" diameter of A3
sketch "Sketch4" plane through (160, 0, 0) normal (1, 0, 0) x (0, 1, 0) in component "Top/Bottom"
  line L0 (7, 10) -> (6, 9)
  line L1 (6, 9) -> (6, 5)
  line L2 (6, 5) -> (3, 5)
  line L3 (3, 5) -> (3, 10)
  line L4 (3, 10) -> (0, 10)
  line L5 (0, 10) -> (0, 0)
  line L6 (0, 0) -> (54, 0)
  line L7 (54, 0) -> (54, 10)
  line L8 (54, 10) -> (51, 10)
  line L9 (51, 10) -> (51, 5)
  line L10 (51, 5) -> (48, 5)
  line L11 (48, 5) -> (48, 9)
  line L12 (48, 9) -> (47, 10)
  line L13 (47, 10) -> (7, 10)
  circle A0 centre (11, 5) radius 1.85
  circle A1 centre (11, 5) radius 1.6
  circle A2 centre (43, 5) radius 1.85
  circle A3 centre (43, 5) radius 1.6
extrude "Extrude5" cut sketch "Sketch4" against normal blind 15 contours A1 | A3 bodies 6 in component "Top/Bottom"
extrude "Extrude6" cut sketch "Sketch4" against normal blind 5 contours A0 | A2 bodies 6 in component "Top/Bottom"
extrude "Extrude7" cut sketch "Sketch3" against normal blind 15 contours A2 | A3 bodies 6 in component "Top/Bottom"
extrude "Extrude8" cut sketch "Sketch3" against normal blind 5 contours A0 | A1 bodies 6 in component "Top/Bottom"
chamfer "Chamfer2''" distance 1 angle 45 4 edges at (0, 44.7248, 5.669) (0, 12.7248, 5.669) (160, 41.2752, 5.669) (160, 9.2752, 5.669) on bodies 6 in component "Top/Bottom"